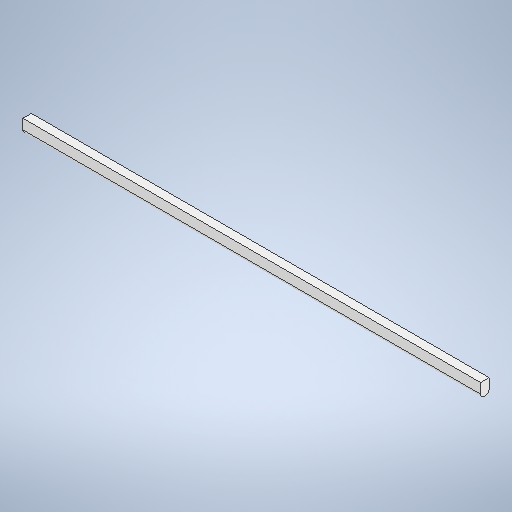
# Autodesk Inventor part: Light tube 118.4cm
Saved by Autodesk Inventor 2025 (Build 290162000, 162)
## iProperties
Created: 2024-06-18
Part Number: Light tube 118.4cm
Material: Generic
Document SubType Name: Modeling
Designer: Isaac
Density: 1 g/cm^3
Appearance: Default
Author: Isaac
Autodesk Inventor part; units mm, degrees
ref_plane "YZ Plane" through (0, 0, 0) normal (1, 0, 0) x (0, 1, 0)
ref_plane "XZ Plane" through (0, 0, 0) normal (0, 1, 0) x (-1, 0, 0)
ref_plane "XY Plane" through (0, 0, 0) normal (0, 0, 1) x (1, 0, 0)
sketch "Sketch1" plane through (0, 0, 0) normal (0, 0, 1) x (1, 0, 0)
  line L0 (-592, 18) -> (592, 18)
  line L1 (592, 18) -> (592, -18)
  line L2 (592, -18) -> (-592, -18)
  line L3 (-592, -18) -> (-592, 18)
  line L4 (-592, 18) -> (592, -18) construction
  line L5 (592, 18) -> (-592, -18) construction
  point P0 (0, 0)
  dimension "d0" = 36
  dimension "d1" = 1184
  constraints: 12 end point, 2 midpoint, 2 parallel, 1 horizontal, 1 perpendicular
  measures "d0" distance of L2.end L0.start
  measures "d1" distance of L0.start L0.end
extrude "Extrusion1" add sketch "Sketch1" along normal blind 22
fillet "Fillet1" radius 10 1 edges at (0, -18, 22)
fillet "Fillet2" radius 10 1 edges at (0, -18, 0)
body "Solid1"
